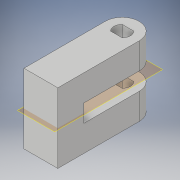
# Autodesk Inventor part: joint_2_part1
Saved by Autodesk Inventor 2019 (Build 230136000, 136)
## iProperties
Created: 2019-12-26
Part Number: joint_2_part1
Material: Типовые
Document SubType Name: Modeling
Designer: Петров Иван
Density: 1 g/cm^3
Appearance: По умолчанию
Author: Петров Иван
Autodesk Inventor part; units mm, degrees
ref_plane "YZ Plane" through (0, 0, 0) normal (1, 0, 0) x (0, 1, 0)
ref_plane "XZ Plane" through (0, 0, 0) normal (0, 1, 0) x (-1, 0, 0)
ref_plane "XY Plane" through (0, 0, 0) normal (0, 0, 1) x (1, 0, 0)
sketch "Эскиз1" plane through (0, 0, 0) normal (0, 1, 0) x (-1, 0, 0)
  arc A0 (6.0208, -6) -> (6.0208, 6) centre (0, 0) ccw
  line L0 (6.0208, -6) -> (-6.0208, -6)
  arc A1 (-6.0208, 6) -> (-6.0208, -6) centre (0, 0) ccw
  line L1 (6.0208, 6) -> (-6.0208, 6)
  line L2 (17.5, 37) -> (-17.5, 37)
  line L3 (-17.5, 37) -> (-17.5, 0)
  arc A2 (-17.5, 0) -> (17.5, 0) centre (0, 0) ccw
  line L4 (17.5, 0) -> (17.5, 37)
  line L5 (17.5, 0) -> (17.5, 57)
  line L6 (-17.5, 37) -> (17.5, 37)
  line L7 (17.5, 37) -> (17.5, 57)
  line L8 (17.5, 57) -> (-17.5, 57)
  line L9 (-17.5, 57) -> (-17.5, 37)
  constraints: 20 end point, 6 point on circle, 3 centre point, 2 parallel, 1 horizontal, 1 perpendicular
extrude "Выдавливание1" add sketch "Эскиз1" along normal blind 27
sketch "Эскиз2" plane through (-17.5, 0, 57) normal (0, 0, 1) x (1, 0, 0)
  line L0 (0, 0) -> (35, 0)
  line L1 (35, 0) -> (35, 72.2)
  line L2 (35, 72.2) -> (0, 72.2)
  line L3 (0, 72.2) -> (0, 0)
  point P0 (17.5, 0)
  dimension "d2" = 72.2
  constraints: 8 end point, 2 parallel, 1 horizontal, 1 perpendicular
  measures "d2" distance of L1.end L0.end
extrude "Выдавливание2" add sketch "Эскиз2" along normal blind 27
ref_plane "РабПлоскость1" through (17.5, 36.1, 84) normal (0, 1, 0) x (1, 0, 0)
mirror "Зеркальное отражение1" about plane through (17.5, 36.1, 84) normal (0, 1, 0) of "Выдавливание1"
